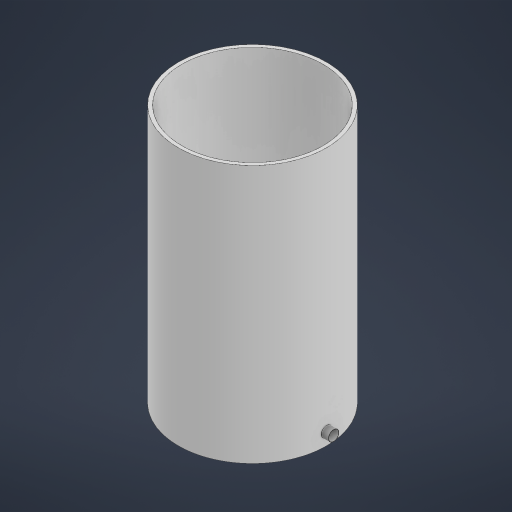
# Autodesk Inventor part: Tank_M
Saved by Autodesk Inventor 2023 (Build 270158000, 158)
## iProperties
Created: 2022-08-20
Part Number: Tank_M
Material: Generic
Document SubType Name: Modeling
Designer: Mike
Density: 1 g/cm^3
Appearance: Default
Author: Mike
Autodesk Inventor part; units mm, degrees
ref_plane "XZ Plane" through (0, 0, 0) normal (0, 1, 0) x (-1, 0, 0)
ref_plane "XY Plane" through (0, 0, 0) normal (0, 0, 1) x (1, 0, 0)
sketch "Sketch1" plane through (0, 0, 0) normal (0, 1, 0) x (-1, 0, 0)
  circle A0 centre (0, 0) radius 200
  circle A1 centre (0, 0) radius 210
  dimension "d0" = 400
  dimension "d1" = 420
  constraints: 2 centre point, 2 coincident
  measures "d0" diameter of A0
  measures "d1" diameter of A1
extrude "Extrusion1" add sketch "Sketch1" against normal blind 10 contours A0 | A1
extrude "Extrusion2" add sketch "Sketch1" along normal blind 721
ref_plane "Work Plane1" through (210, 0, 0) normal (1, 0, 0) x (0, 1, 0)
sketch "Sketch2" plane through (210, 0, 0) normal (1, 0, 0) x (0, 1, 0)
  circle A0 centre (25, 0) radius 15
  point P0 (0, 0)
  dimension "d7" = 30
  dimension "d8" = 25
  constraints: 1 centre point
  measures "d7" diameter of A0
  measures "d8" distance of point (0, 0) A0.centre
hole "Hole1" at (210, 25, 0) direction (-1, 0, 0) diameter 30 depth 22 tip angle 118
thread "Thread1" size "M30x3.5" class "6H" standard "ANSI Metric M Profile" full length
extrude "Extrusion3" add sketch "Sketch2" along normal blind 20
sketch "Sketch3" plane through (230, 25, 0) normal (1, 0, 0) x (0, 0, -1)
  circle A0 centre (0, 0) radius 14.175
  point P0 (0, -25)
  dimension "d20" = 28.35
  constraints: 1 centre point
  measures "d20" diameter of A0
extrude "Extrusion4" cut sketch "Sketch3" against normal blind 20
body "Solid1"
